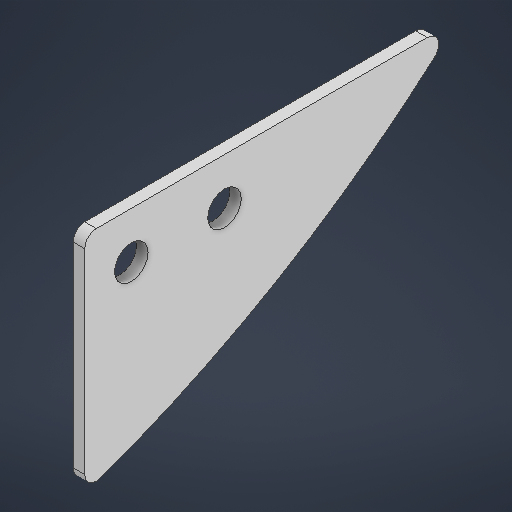
# Autodesk Inventor part: hg
Saved by Autodesk Inventor 2025.2 (Build 292293000, 293)
## iProperties
Created: 2025-04-17
Part Number: hg
Material: Generic
Document SubType Name: Modeling
Designer: roejo
Density: 1 g/cm^3
Appearance: Default
Author: roejo
Autodesk Inventor part; units mm, degrees
ref_plane "YZ Plane" through (0, 0, 0) normal (1, 0, 0) x (0, 1, 0)
ref_plane "XZ Plane" through (0, 0, 0) normal (0, 1, 0) x (-1, 0, 0)
ref_plane "XY Plane" through (0, 0, 0) normal (0, 0, 1) x (1, 0, 0)
sketch "Sketch1" plane through (0, 0, 0) normal (1, 0, 0) x (0, 1, 0)
  line L0 (2.2349, 0) -> (28.8925, 0)
  line L1 (30.48, 0) -> (24.13, 0)
  circle A0 centre (24.13, -6.35) radius 2.286
  circle A1 centre (24.13, -19.05) radius 2.286
  line L2 (30.48, -1.5875) -> (30.48, -46.6985)
  arc A2 (30.48, -1.5875) -> (28.8925, 0) centre (28.8925, -1.5875) ccw
  arc A3 (0.7402, -2.1223) -> (27.703, -47.7499) centre (132.7707, 45.1184) ccw
  arc A4 (27.703, -47.7499) -> (30.48, -46.6985) centre (28.8925, -46.6985) ccw
  arc A5 (2.2349, 0) -> (0.7402, -2.1223) centre (2.2349, -1.5875) ccw
  point P0 (0, 0)
  point P1 (30.48, -38.1)
  point P2 (30.48, -38.1)
  point P3 (30.48, -38.1)
  point P4 (30.48, -38.1)
  point P5 (0, 0)
  point P6 (0, 0)
  point P7 (0, 0)
  point P8 (30.48, -38.1)
  point P9 (30.48, -38.1)
  point P10 (30.48, -38.1)
  point P11 (0, 0)
  point P12 (0, 0)
  point P13 (0, 0)
  point P14 (30.48, -50.8)
  point P15 (0, 0)
  point P16 (0, 0)
  point P17 (0, 0)
  point P18 (30.48, -50.8)
  point P19 (30.48, -50.8)
  point P20 (30.48, -50.8)
  dimension "d0" = 30.48
  dimension "d1" = 38.1
  dimension "d6" = 4.572
  dimension "d7" = 4.572
  dimension "d10" = 50.8
  dimension "d13" = 1.5875
  dimension "d16" = 1.5875
  constraints: 10 point on circle, 9 point on line, 6 centre point, 6 end point, 6 tangent, 4 horizontal, 1 equal radius, 1 perpendicular, 1 vertical, 24 other
  measures "d0" distance of point (0, 0) L1.start
  measures "d1" distance of L1.start point (30.48, -38.1)
  measures "d6" diameter of A0
  measures "d7" diameter of A1
  measures "d10" distance of L1.start point (30.48, -50.8)
  measures "d13" radius of A2
  measures "d16" radius of A4
extrude "Extrusion1" add sketch "Sketch1" along normal blind 1.5875
body "Solid1"
